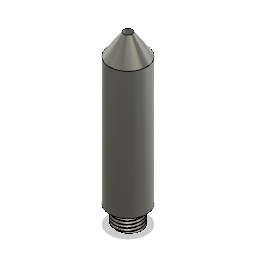
probeTop (Autodesk Fusion 360 design; units mm, degrees)
Autodesk Fusion 360 part; units mm, degrees
sketch "Sketch1" plane through (0, 0, 0) normal (0, 1, 0) x (1, 0, 0)
  circle A0 centre (0, 0) radius 8.75
  dimension "d1" = 17.5
  measures "d1" diameter of A0
extrude "Extrude1" add sketch "Sketch1" along normal blind 68 makes body 1
ref_plane "WorkPlane1" through (0, 78, 0) normal (0, 1, 0) x (1, 0, 0)
sketch "Sketch2" plane through (0, 78, 0) normal (0, 1, 0) x (1, 0, 0)
  circle A0 centre (0, 0) radius 2
  dimension "d5" = 4
  measures "d5" diameter of A0
loft "Loft1" add profiles "Sketch2" section 1 section 2 face at (2.2113, 68, 2.9606) on bodies 1 bodies 1
extrude "Extrude2" cut 1 faces at (0.637, 78, -0.1965) along direction (0, -1, 0) blind 78 on bodies 1 bodies 1
split "Split1" by plane through (0, 8, 0) normal (0, -1, 0) bodies 1 makes body 2 at (8.7065, 5.3333, -0.8712)
thread "Thread1" "ANSI Unified Screw Threads 0.5 1/2-18 UNS 2A" major diameter 12.5578 minor diameter 10.988 pitch 1.4111 angle 60 modelled right hand crest width 0.1764 on face at (8.7065, 5.3333, -0.8712) crest through (6.2789, -0.0882, 0) on bodies 2
combine "Combine1" operation add target body 2 tool bodies 1
